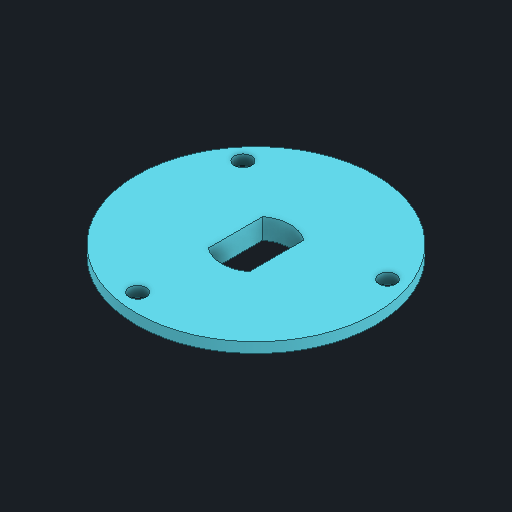
# Autodesk Inventor part: tibea_vodilo_steel
Saved by Autodesk Inventor 2026 (Build 300175000, 175)
## iProperties
Created: 2026-04-25
Part Number: tibea_vodilo_steel
Material: Сталь
Document SubType Name: Modeling
Designer: user
Density: 7.85 g/cm^3
Appearance: Серо-синий
Mass: 101.318 g
Surface Area: 86.0711 cm^2
Volume: 12.9068 cm^3
Author: user
Autodesk Inventor part; units mm, degrees
ref_plane "YZ Plane" through (0, 0, 0) normal (1, 0, 0) x (0, 1, 0)
ref_plane "XZ Plane" through (0, 0, 0) normal (0, 1, 0) x (-1, 0, 0)
ref_plane "XY Plane" through (0, 0, 0) normal (0, 0, 1) x (1, 0, 0)
sketch "Эскиз1" plane through (0, 0, 0) normal (0, 1, 0) x (-1, 0, 0)
  line L0 (48.4444, -60.6419) -> (48.4444, -44.6419) projected
  arc A0 (60.4444, -44.6419) -> (48.4444, -44.6419) centre (54.4444, -52.6419) ccw projected
  line L1 (60.4444, -44.6419) -> (60.4444, -60.6419) projected
  arc A1 (48.4444, -60.6419) -> (60.4444, -60.6419) centre (54.4444, -52.6419) ccw projected
  circle A2 centre (54.4444, -52.6419) radius 30 construction
  circle A3 centre (54.4444, -52.6419) radius 35
  circle A4 centre (26.286, -62.9913) radius 2.5
  circle A5 centre (54.4444, -52.6419) radius 30 construction
  circle A6 centre (77.4863, -71.8531) radius 2.5
  circle A7 centre (54.4444, -52.6419) radius 30 construction
  circle A8 centre (59.5607, -23.0814) radius 2.5
  point P0 (0, 0)
  point P1 (109.6501, -75.8137)
  dimension "d5" = 60
  dimension "d4" = 70
  dimension "d6" = 5
  dimension "d9" = 360
  constraints: 4 centre point, 2 coincident, 22 other
  measures "d4" diameter of A3
  measures "d6" diameter of A4
extrude "Выдавливание1" add sketch "Эскиз1" along normal blind 3
sketch "Эскиз4" plane through (-54.4444, 0, -52.6419) normal (0, -1, 0) x (1, 0, 0)
  circle A0 centre (0, 0) radius 35 projected
  circle A1 centre (-5.1164, 29.5605) radius 2.5 projected
  circle A2 centre (-23.042, -19.2112) radius 2.5 projected
  circle A3 centre (28.1583, -10.3493) radius 2.5 projected
  line L0 (-6, 8) -> (-6, -8) projected
  arc A4 (6, 8) -> (-6, 8) centre (0, 0) ccw projected
  line L1 (6, -8) -> (6, 8) projected
  arc A5 (-6, -8) -> (6, -8) centre (0, 0) ccw projected
  circle A6 centre (0, 0) radius 17.5
  point P0 (54.4444, 52.6419)
  dimension "d14" = 35
  constraints: 1 centre point, 1 coincident
  measures "d14" diameter of A6
extrude "Выдавливание3" add sketch "Эскиз4" along normal blind 3 contours A6
equation "\"d2\" = thickness_steel"
equation "\"d15\" = thickness_steel"
equation "\"tolerance_plazma\" = 0.1"
equation "\"thickness_steel\" = 3"
equation "\"d_main_screw_holes\" = 6.1"
equation "\"thickness_profile_tibea\" = 4"
equation "\"thickness_profile_femur\" = 3"
equation "\"width_shaft_shift\" = 35"
equation "\"width_flattened_surface\" = 12"
